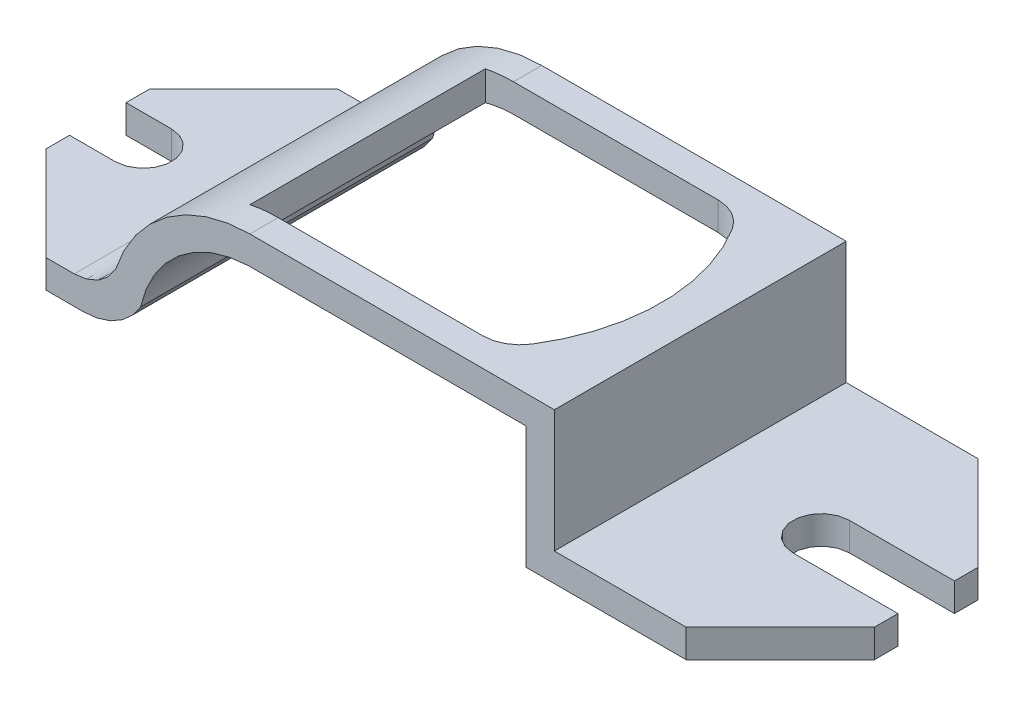
# Autodesk Inventor part: SUPPORT PLSTE
Saved by Autodesk Inventor 2014 (Build 180170000, 170)
## iProperties
Created: 2014-12-12
Part Number: SUPPORT PLSTE
Material: Stainless Steel, 440C
Document SubType Name: Modeling
Designer: Ebrahim
Density: 7.75 g/cm^3
Appearance: Semi-Polished
Mass: 52.8516 g
Surface Area: 56.7684 cm^2
Volume: 6.81956 cm^3
Author: Ebrahim
Autodesk Inventor part; units mm, degrees
ref_plane "YZ Plane" through (0, 0, 0) normal (1, 0, 0) x (0, 1, 0)
ref_plane "XZ Plane" through (0, 0, 0) normal (0, 1, 0) x (-1, 0, 0)
ref_plane "XY Plane" through (0, 0, 0) normal (0, 0, 1) x (1, 0, 0)
sketch "Sketch8" plane through (0, 0, 0) normal (0, 0, 1) x (1, 0, 0)
  line L0 (26.5434, 0) -> (-0.4566, 0)
  line L1 (-0.4566, 0) -> (-0.4566, 13)
  line L2 (-47.4566, 0) -> (-61.4566, 0)
  line L3 (-61.4566, 3) -> (-48.4566, 3)
  line L4 (-29.793, 16) -> (2.5434, 16)
  line L5 (2.5434, 16) -> (2.5434, 3)
  line L6 (2.5434, 3) -> (26.5434, 3)
  line L7 (-61.4566, 0) -> (-61.4566, 3)
  line L8 (26.5434, 3) -> (26.5434, 0)
  line L9 (-29.4566, 30.4084) -> (-29.4566, -16.4271)
  arc A0 (-29.4566, 13) -> (-30.0706, 12.9895) centre (-29.4566, -5) ccw
  arc A1 (-30.0706, 12.9895) -> (-41.3988, 3.4923) centre (-29.6612, 0.9965) ccw
  arc A2 (-48.4566, 3) -> (-44.0702, 5.6) centre (-48.4566, 8) ccw
  line L10 (-0.4566, 13) -> (-29.4566, 13)
  arc A3 (-47.4566, 0) -> (-41.3988, 3.4923) centre (-47.4566, 7) ccw
  arc A4 (-29.793, 16) -> (-44.0702, 5.6) centre (-29.793, 1) ccw
  point P0 (0, 0)
  point P1 (-36.7292, 11.4654)
  point P2 (-29.4566, -11.7979)
  dimension "d92" = 88
  dimension "d93" = 27
  dimension "d95" = 16
  dimension "d100" = 3
  dimension "d101" = 3
  dimension "d104" = 14
  dimension "d105" = 13
  dimension "d106" = 32
  dimension "d109" = 5
  dimension "d111" = 12
  dimension "d112" = 7
  dimension "d113" = 3
  dimension "d114" = 15
  constraints: 22 end point, 11 point on circle, 5 centre point, 5 tangent, 4 parallel, 3 collinear, 3 perpendicular, 3 point on line, 1 horizontal, 1 other
  measures "d92" distance between parallel lines of L7 L8
  measures "d93" distance between parallel lines of L1 L8
  measures "d95" distance between parallel lines of L0 L4
  measures "d100" distance between parallel lines of L2 L3
  measures "d101" distance of L6.end L0.start
  measures "d104" distance of L2.start L2.end
  measures "d105" distance of L3.start L3.end
  measures "d106" distance between parallel lines of L7 L9
  measures "d109" radius of A2
  measures "d111" radius of A1
  measures "d112" radius of A3
  measures "d113" distance between parallel lines of L10 L4
  measures "d114" radius of A4
extrude "Extrusion8" add sketch "Sketch8" along normal mid plane 31
sketch "Sketch9" plane through (-29.793, 16, 15.5) normal (0, 1, 0) x (1, 0, 0)
  line L0 (0, 0) -> (0, 31) projected
  line L1 (32.3364, 0) -> (0, 0) projected
  line L2 (0, 31) -> (32.3364, 31) projected
  arc A0 (8.6831, 6.377) -> (8.6831, 24.0275) centre (7.7775, 15.2022) ccw construction
  line L3 (-3, 28) -> (-3, 3)
  line L4 (-3, 28) -> (21.7382, 28)
  line L5 (-3, 3) -> (21.7382, 3)
  arc A1 (25.1271, 4.875) -> (25.1271, 26.125) centre (8.1828, 15.5) ccw
  arc A2 (25.1271, 26.125) -> (21.7382, 28) centre (21.7382, 24) ccw
  arc A3 (21.7382, 3) -> (25.1271, 4.875) centre (21.7382, 7) ccw
  point P0 (29.793, 15.5)
  point P1 (23.7953, 28)
  point P2 (23.7953, 3)
  dimension "d115" = 3
  dimension "d116" = 3
  dimension "d117" = 3
  dimension "d118" = 20
  dimension "d119" = 4
  constraints: 8 point on circle, 6 end point, 4 tangent, 3 centre point, 2 perpendicular, 2 point on line, 1 equal radius, 1 parallel
  measures "d115" distance between parallel lines of L4 L2
  measures "d116" distance between parallel lines of L5 L1
  measures "d117" distance between parallel lines of L3 L0
  measures "d118" radius of A1
  measures "d119" radius of A2
extrude "Extrusion9" cut sketch "Sketch9" against normal blind 4
sketch "Sketch10" plane through (2.5434, 3, 15.5) normal (0, 1, 0) x (1, 0, 0)
  line L0 (24, 0) -> (24, 31) projected
  line L1 (0, 31) -> (24, 31) projected
  circle A0 centre (12.8467, 12.1299) radius 2.4585 projected
  circle A1 centre (-59.1533, 12.1299) radius 2.4585 projected
  line L2 (24, 15.5) -> (-63.997, 15.5) construction
  line L3 (12.8467, 12.1299) -> (12.8467, 22.8922)
  line L4 (-59.1533, 12.1299) -> (-59.1533, 22.8922)
  point P0 (-2.5434, 15.5)
  point P1 (-59.1533, 15.5)
  point P2 (12.8467, 15.5)
  constraints: 6 end point, 4 point on line, 2 parallel, 1 midpoint, 1 perpendicular
hole "Hole1" at (-56.6099, 3, 0) at (15.3901, 3, 0) direction (0, -1, 0) diameter 6 depth 5 tip angle 118
sketch "Sketch11" plane through (2.5434, 3, 15.5) normal (0, 1, 0) x (1, 0, 0)
  circle A0 centre (12.8467, 15.5) radius 3 projected
  line L0 (24, 0) -> (0, 0) projected
  line L1 (12.8467, 15.5) -> (37.9107, 15.5) construction
  line L2 (12.8467, 12.5) -> (37.9107, 12.5)
  line L3 (37.9107, 18.5) -> (12.8467, 18.5)
  arc A1 (12.8467, 18.5) -> (12.8467, 12.5) centre (12.8467, 15.5) ccw
  arc A2 (37.9107, 12.5) -> (37.9107, 18.5) centre (37.9107, 15.5) ccw
  circle A3 centre (-59.1533, 15.5) radius 3 projected
  line L4 (-59.1533, 15.5) -> (-73.4296, 15.5) construction
  line L5 (-59.1533, 12.5) -> (-73.4296, 12.5)
  line L6 (-73.4296, 18.5) -> (-59.1533, 18.5)
  arc A4 (-59.1533, 12.5) -> (-59.1533, 18.5) centre (-59.1533, 15.5) ccw
  arc A5 (-73.4296, 18.5) -> (-73.4296, 12.5) centre (-73.4296, 15.5) ccw
  point P0 (-2.5434, 15.5)
  point P1 (25.3787, 15.5)
  point P2 (-66.2914, 15.5)
  constraints: 16 end point, 8 point on circle, 8 tangent, 4 centre point, 4 parallel, 2 concentric, 2 midpoint
extrude "Extrusion10" cut sketch "Sketch11" against normal blind 4 contours A0 L3 A2 L2 | A3 | A3 L5 A5 L6
chamfer "Chamfer1" distance 10 angle 45 4 edges at (26.5434, 1.5, 15.5) (-61.4566, 1.5, 15.5) (-61.4566, 1.5, -15.5) (26.5434, 1.5, -15.5)
equation "\"d2\" = 0.5 * d1"
equation "\"d3\" = 0.5 * d0"
equation "\"d1\" = 33"
equation "\"d0\" = 94.155"
body "Solid2"
